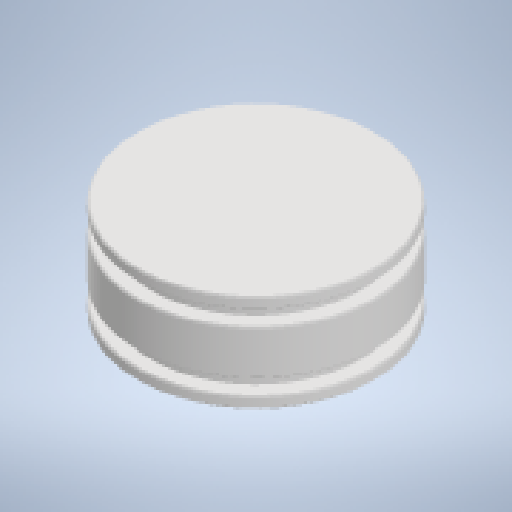
# Autodesk Inventor part: 2 Piston
Saved by Autodesk Inventor 2024 (Build 280153000, 153)
## iProperties
Created: 2024-04-17
Part Number: 2 Piston
Material: Generic
Document SubType Name: Modeling
Designer: Tommy Rohmann
Density: 1 g/cm^3
Appearance: Default
Author: Tommy Rohmann
Autodesk Inventor part; units mm, degrees
ref_plane "YZ Plane" through (0, 0, 0) normal (1, 0, 0) x (0, 1, 0)
ref_plane "XZ Plane" through (0, 0, 0) normal (0, 1, 0) x (-1, 0, 0)
ref_plane "XY Plane" through (0, 0, 0) normal (0, 0, 1) x (1, 0, 0)
sketch "Sketch1" plane through (0, 0, 0) normal (0, 0, 1) x (1, 0, 0)
  line L0 (50.8, 0) -> (50.8, 39.0312) construction
  line L1 (0, 0) -> (50.6412, 0)
  line L2 (44.45, 0) -> (44.45, 51.6727)
  line L3 (0, 0) -> (0, 50.5742)
  line L4 (50.6412, 0) -> (50.6412, 45.6895)
  line L5 (50.6412, 4.7625) -> (44.45, 4.7625)
  line L6 (44.45, 11.1125) -> (50.6412, 11.1125)
  line L7 (50.6412, 30.1625) -> (44.45, 30.1625)
  line L8 (44.45, 36.5125) -> (50.6412, 36.5125)
  line L9 (50.6412, 41.275) -> (0, 41.275)
  point P0 (47.5456, 36.5125)
  point P1 (44.45, 30.1625)
  dimension "d1" = 50.6412
  dimension "d2" = 44.45
  dimension "d3" = 6.35
  dimension "d4" = 6.35
  dimension "d5" = 4.7625
  dimension "d6" = 19.05
  dimension "d7" = 4.7625
  dimension "d12" = 41.275
  constraints: 20 end point, 10 point on line, 3 vertical, 2 horizontal, 2 perpendicular, 1 midpoint
  measures "d1" distance of L1.start L1.end
  measures "d2" distance between parallel lines of L2 L3
  measures "d3" distance from line of point (47.546, 36.513) L7
  measures "d4" distance between parallel lines of L5 L6
  measures "d5" distance between parallel lines of L1 L5
  measures "d6" distance between parallel lines of L6 L7
  measures "d7" distance between parallel lines of L8 L9
  measures "d12" distance between parallel lines of L9 L1
revolve "Revolution1" add sketch "Sketch1" angle 360 about axis through (0, 0, 0) along (0, 1, 0) contours L3 L9 L2 L1 | L2 L5 L4 L1 | L9 L4 L8 L2 | L2 L7 L4 L6
chamfer "Chamfer1" distance 0.635 angle 45 6 edges at (-50.6412, 0, 0) (-50.6412, 4.7625, 0) (-50.6412, 11.1125, 0) (-50.6412, 30.1625, 0) (-50.6412, 36.5125, 0) (-50.6412, 41.275, 0)
sketch "Sketch2" plane through (0, 0, 0) normal (0, -1, 0) x (1, 0, 0)
  circle A0 centre (0, 0) radius 9.7409
  circle A1 centre (0, 0) radius 11.1125
  dimension "d16" = 19.4818
  dimension "d17" = 22.225
  constraints: 2 centre point, 2 coincident
  measures "d16" diameter of A0
  measures "d17" diameter of A1
extrude "Extrusion1" cut sketch "Sketch2" against normal up to surface (30.1625 mm away) contours A0
extrude "Extrusion2" cut sketch "Sketch2" against normal blind 6.35 contours A0 | A1
equation "\"MachineMaxHeight\" = 539.75"
equation "\"MachineMaxWidth\" = 215.9"
equation "\"MachineMaxLength\" = 266.7"
equation "\"MachineFluidCapacity\" = 25.4"
equation "\"MaxCompressiveCapacity\" = 20320"
equation "\"WashChamberID\" = 101.6"
equation "\"WashChamberOD\" = 114.3"
equation "\"ConduitThickness\" = 152.4"
equation "\"SealedSurfaceOffset\" = 0.15875"
equation "\"StaticORingThickness\" = 4.7625"
body "Solid1"
